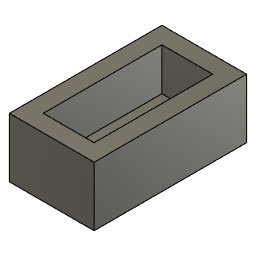
holder (Autodesk Fusion 360 design; units mm, degrees)
Autodesk Fusion 360 part; units mm, degrees
sketch "Sketch1" plane through (0, 0, 0) normal (0, 1, 0) x (1, 0, 0)
  line L0 (0, 0) -> (6, 0)
  line L1 (6, 0) -> (6, 14)
  line L2 (6, 14) -> (0, 14)
  line L3 (0, 14) -> (0, 0)
  line L4 (-2, 16) -> (8, 16)
  line L5 (8, 16) -> (8, 0)
  line L6 (8, 0) -> (8, -2)
  line L7 (8, -2) -> (-2, -2)
  line L8 (-2, -2) -> (-2, 16)
  dimension "d1" = 6
  dimension "d2" = 14
  constraint horizontal L0
  constraint vertical L1
  constraint horizontal L2
  constraint vertical L3
  constraint coincident L0.start L3.end
  constraint horizontal L4
  constraint perpendicular L4 L5
  constraint parallel L5 L6
  constraint perpendicular L6 L7
  constraint perpendicular L7 L8
  measures "d1" distance of L0.start L0.end
  measures "d2" distance of L0.start L2.end
extrude "Extrude1" add sketch "Sketch1" along normal blind 5
sketch "Sketch2" plane through (0, 0, 0) normal (0, 1, 0) x (1, 0, 0)
  line L0 (8, 16) -> (-2, 16)
  line L1 (-2, 16) -> (-2, -2)
  line L2 (-2, -2) -> (8, -2)
  line L3 (8, -2) -> (8, 16)
  line L4 (5, 13) -> (1, 13)
  line L5 (1, 13) -> (1, 1)
  line L6 (1, 1) -> (5, 1)
  line L7 (5, 1) -> (5, 13)
  line L8 (8, 16) -> (8, -2)
  line L9 (-2, -2) -> (8, -2)
  line L10 (-2, -2) -> (-2, 16)
  line L11 (8, 16) -> (-2, 16)
  constraint horizontal L0
  constraint vertical L1
  constraint horizontal L2
  constraint vertical L3
  constraint horizontal L4
  constraint perpendicular L4 L5
  constraint perpendicular L5 L6
  constraint perpendicular L4 L7
extrude "Extrude2" add sketch "Sketch2" against normal blind 2
